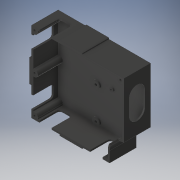
# Autodesk Inventor part: electronics_compartement
Saved by Autodesk Inventor 2019.4 (Build 234330000, 330)
## iProperties
Created: 2020-10-28
Part Number: electronics_compartement
Material: Generic
Document SubType Name: Modeling
Designer: deanv
Density: 1 g/cm^3
Appearance: Smooth - Black
Author: deanv
Autodesk Inventor part; units mm, degrees
ref_plane "YZ Plane" through (0, 0, 0) normal (1, 0, 0) x (0, 1, 0)
ref_plane "XZ Plane" through (0, 0, 0) normal (0, 1, 0) x (-1, 0, 0)
ref_plane "XY Plane" through (0, 0, 0) normal (0, 0, 1) x (1, 0, 0)
sketch "Sketch1" plane through (0, 0, 0) normal (0, 0, 1) x (1, 0, 0)
  line L0 (-73.5, 64) -> (73.5, 64)
  line L1 (73.5, 64) -> (73.5, -64)
  line L2 (73.5, -64) -> (-73.5, -64)
  line L3 (-73.5, -64) -> (-73.5, 64)
  line L4 (-73.5, 64) -> (73.5, -64) construction
  line L5 (73.5, 64) -> (-73.5, -64) construction
  line L6 (71, -61.5) -> (-71, -61.5)
  line L7 (-71, -61.5) -> (-71, 61.5)
  line L8 (-71, 61.5) -> (71, 61.5)
  line L9 (71, 61.5) -> (71, -61.5)
  line L10 (71, -61.5) -> (-71, 61.5) construction
  line L11 (-71, -61.5) -> (71, 61.5) construction
  line L12 (-73.5, 18.5) -> (-76.5, 18.5)
  line L13 (-76.5, 18.5) -> (-76.5, -18.5)
  line L14 (-76.5, -18.5) -> (-73.5, -18.5)
  line L15 (-73.5, -18.5) -> (-73.5, 18.5)
  line L16 (-73.5, 0) -> (73.5, 0) construction
  line L17 (0, -64) -> (0, 64) construction
  line L18 (-28.5, 64) -> (7.5, 64)
  line L19 (7.5, 64) -> (7.5, 66)
  line L20 (7.5, 66) -> (-28.5, 66)
  line L21 (-28.5, 66) -> (-28.5, 64)
  line L22 (-28.5, -64) -> (7.5, -64)
  line L23 (7.5, -64) -> (7.5, -66)
  line L24 (7.5, -66) -> (-28.5, -66)
  line L25 (-28.5, -66) -> (-28.5, -64)
  line L26 (73.5, -64) -> (51, -64) construction
  line L27 (51, -64) -> (51, -24.6) construction
  line L28 (51, -24.6) -> (73.5, -24.6) construction
  line L29 (73.5, -24.6) -> (73.5, -64) construction
  line L30 (51, -24.6) -> (73.5, -24.6) construction
  line L31 (73.5, -24.6) -> (73.5, -47.1) construction
  line L32 (73.5, -47.1) -> (51, -47.1) construction
  line L33 (51, -47.1) -> (51, -24.6) construction
  arc A0 (73.5, -24.6) -> (51, -47.1) centre (73.5, -47.1) ccw
  line L34 (51, -47.1) -> (51, -64)
  line L35 (73.5, -47.1) -> (48.5, -47.1) construction
  line L36 (48.5, -47.1) -> (48.5, -22.1) construction
  line L37 (48.5, -22.1) -> (73.5, -22.1) construction
  line L38 (73.5, -22.1) -> (73.5, -47.1) construction
  arc A1 (73.5, -22.1) -> (48.5, -47.1) centre (73.5, -47.1) ccw
  line L39 (48.5, -47.1) -> (48.5, -64)
  line L40 (-73.5, -64) -> (-68.5, -64) construction
  line L41 (-68.5, -64) -> (-68.5, -59) construction
  line L42 (-68.5, -59) -> (-73.5, -59) construction
  line L43 (-73.5, -59) -> (-73.5, -64) construction
  circle A2 centre (-68.5, -59) radius 5
  line L44 (-68.5, -54) -> (-73.5, -54)
  line L45 (-63.5, -59) -> (-63.5, -64)
  line L46 (-73.5, 64) -> (-68.5, 64) construction
  line L47 (-68.5, 64) -> (-68.5, 59) construction
  line L48 (-68.5, 59) -> (-73.5, 59) construction
  line L49 (-73.5, 59) -> (-73.5, 64) construction
  circle A3 centre (-68.5, 59) radius 5
  line L50 (-68.5, 54) -> (-73.5, 54)
  line L51 (-63.5, 59) -> (-63.5, 64)
  line L52 (-71, -1.25) -> (-68.5, -1.25) construction
  line L53 (-68.5, -1.25) -> (-68.5, 1.25) construction
  line L54 (-68.5, 1.25) -> (-71, 1.25) construction
  line L55 (-71, 1.25) -> (-71, -1.25) construction
  circle A4 centre (-68.5, 0) radius 5
  line L56 (-68.5, 5) -> (-73.5, 5)
  line L57 (-68.5, -5) -> (-73.5, -5)
  arc A5 (73.5, -24.6) -> (51, -47.1) centre (73.5, -47.1) ccw
  line L58 (51, -47.1) -> (51, -64)
  line L59 (51, -64) -> (73.5, -64)
  line L60 (73.5, -64) -> (73.5, -24.6)
  line L61 (71, 61.5) -> (-71, 61.5)
  line L62 (-71, 61.5) -> (-71, -61.5)
  line L63 (-71, -61.5) -> (71, -61.5)
  line L64 (71, -61.5) -> (71, 61.5)
  line L65 (71, 61.5) -> (-71, -61.5) construction
  line L66 (-71, 61.5) -> (71, -61.5) construction
  line L67 (73.5, 64) -> (-73.5, 64)
  line L68 (-73.5, 64) -> (-73.5, -64)
  line L69 (-73.5, -64) -> (73.5, -64)
  line L70 (73.5, -64) -> (73.5, 64)
  line L71 (73.5, 64) -> (-73.5, -64) construction
  line L72 (-73.5, 64) -> (73.5, -64) construction
  line L73 (-73.5, 64) -> (73.5, 64)
  line L74 (73.5, 64) -> (73.5, -64)
  line L75 (73.5, -64) -> (-73.5, -64)
  line L76 (-73.5, -64) -> (-73.5, 64)
  line L77 (71, -61.5) -> (-71, -61.5)
  line L78 (-71, -61.5) -> (-71, 61.5)
  line L79 (-71, 61.5) -> (71, 61.5)
  line L80 (71, 61.5) -> (71, -61.5)
  arc A6 (73.5, -24.6) -> (51, -47.1) centre (73.5, -47.1) ccw
  arc A7 (73.5, -22.1) -> (48.5, -47.1) centre (73.5, -47.1) ccw
  line L81 (73.5, -22.1) -> (73.5, -24.6)
  line L82 (51, -47.1) -> (51, -64)
  line L83 (51, -64) -> (48.5, -64)
  line L84 (48.5, -64) -> (48.5, -47.1)
  line L85 (73.5, 64) -> (68.5, 64) construction
  line L86 (68.5, 64) -> (68.5, 59) construction
  line L87 (68.5, 59) -> (73.5, 59) construction
  line L88 (73.5, 59) -> (73.5, 64) construction
  circle A8 centre (68.5, 59) radius 5
  line L89 (63.5, 59) -> (63.5, 64)
  line L90 (68.5, 54) -> (73.5, 54)
  circle A9 centre (17.2, 49) radius 3.25
  circle A10 centre (68, 33.777) radius 3.25
  circle A11 centre (68, 5.837) radius 3.25
  circle A12 centre (15.93, 0.757) radius 3.25
  circle A13 centre (17.2, 49) radius 3.25
  circle A14 centre (68, 33.777) radius 3.25
  circle A15 centre (68, 5.837) radius 3.25
  circle A16 centre (15.93, 0.757) radius 3.25
  line L91 (-33.5, -61.5) -> (16.5, -61.5) construction
  line L92 (16.5, -61.5) -> (16.5, 1.5) construction
  line L93 (16.5, 1.5) -> (-33.5, 1.5) construction
  line L94 (-33.5, 1.5) -> (-33.5, -61.5) construction
  line L95 (-33.5, -61.5) -> (16.5, 1.5) construction
  line L96 (16.5, -61.5) -> (-33.5, 1.5) construction
  line L97 (16.5, -51.5) -> (-33.5, -51.5) construction
  line L98 (-33.5, -51.5) -> (-33.5, -8.5) construction
  line L99 (-33.5, -8.5) -> (16.5, -8.5) construction
  line L100 (16.5, -8.5) -> (16.5, -51.5) construction
  line L101 (16.5, -51.5) -> (-33.5, -8.5) construction
  line L102 (-33.5, -51.5) -> (16.5, -8.5) construction
  line L103 (-8.5, 1.5) -> (-8.5, -61.5) construction
  circle A17 centre (-8.5, -4.5) radius 6
  circle A18 centre (-8.5, -55.5) radius 6
  point P0 (0, 0)
  point P1 (-8.5, -30)
  point P2 (0, -61.5)
  dimension "d130" = 12
  dimension "d131" = 12
  dimension "d0" = 147
  dimension "d1" = 128
  dimension "d7" = 37
  dimension "d8" = 18.5
  dimension "d9" = 3
  dimension "d10" = 2
  dimension "d11" = 36
  dimension "d12" = 45
  dimension "d13" = 2
  dimension "d14" = 36
  dimension "d15" = 45
  dimension "d16" = 22.5
  dimension "d17" = 39.4
  dimension "d18" = 22.5
  dimension "d19" = 22.5
  dimension "d20" = 142
  dimension "d21" = 123
  dimension "d22" = 25
  dimension "d23" = 25
  dimension "d24" = 25
  dimension "d25" = 5
  dimension "d26" = 5
  dimension "d27" = 5
  dimension "d28" = 5
  dimension "d29" = 2.5
  dimension "d30" = 2.5
  dimension "d31" = 1.25
  dimension "d92" = 5
  dimension "d93" = 5
  dimension "d105" = 27.94
  dimension "d106" = 52.07
  dimension "d107" = 48.243
  dimension "d108" = 50.8
  dimension "d109" = 1.27
  dimension "d110" = 5.08
  dimension "d111" = 3
  dimension "d112" = 12.5
  dimension "d113" = 6.5
  dimension "d114" = 6.5
  dimension "d115" = 6.5
  dimension "d116" = 6.5
  dimension "d126" = 63
  dimension "d127" = 50
  dimension "d128" = 50
  dimension "d129" = 43
  dimension "d132" = 37.5
  constraints: 208 end point, 37 parallel, 30 perpendicular, 21 point on circle, 20 midpoint, 18 horizontal, 17 centre point, 17 point on line, 13 coincident, 9 tangent, 7 concentric, 3 collinear, 2 vertical alignment, 4 other
  measures "d0" distance of L1.end L2.end
  measures "d1" distance of L0.end L1.end
  measures "d7" distance between parallel lines of L12 L14
  measures "d8" distance between parallel lines of L16 L12
  measures "d9" distance between parallel lines of L3 L13
  measures "d10" distance between parallel lines of L2 L24
  measures "d11" distance between parallel lines of L23 L25
  measures "d12" distance between parallel lines of L3 L25
  measures "d13" distance of L20.end L18.start
  measures "d14" distance of L19.end L20.end
  measures "d15" distance between parallel lines of L3 L21
  measures "d16" distance of L27.end L28.end
  measures "d17" distance of L26.end L27.end
  measures "d18" distance between parallel lines of L28 L32
  measures "d19" radius of A0
  measures "d20" distance of L6.start L6.end
  measures "d21" distance of L8.end L6.start
  measures "d22" distance of L36.end L37.end
  measures "d23" distance of L35.end L36.end
  measures "d24" radius of A1
  measures "d25" distance of L42.end L41.end
  measures "d26" distance of L41.end L40.end
  measures "d27" distance of L47.end L48.end
  measures "d28" distance of L46.end L47.end
  measures "d29" distance of L53.end L54.end
  measures "d30" distance of L52.end L53.end
  measures "d31" distance between parallel lines of L16 L54
  measures "d92" distance of L87.end L86.end
  measures "d93" distance of L86.end L85.end
  measures "d105" distance of point (68, 33.777) point (68, 5.837)
  measures "d106" horizontal distance of point (15.93, 0.757) point (68, 5.837)
  measures "d107" vertical distance of point (17.2, 49) point (15.93, 0.757)
  measures "d108" horizontal distance of point (68, 33.777) point (17.2, 49)
  measures "d109" horizontal distance of point (17.2, 49) point (15.93, 0.757)
  measures "d110" vertical distance of point (68, 5.837) point (15.93, 0.757)
  measures "d111" distance from line of L9 point (68, 5.837)
  measures "d112" distance from line of L8 point (17.2, 49)
  measures "d113" diameter of A9
  measures "d114" diameter of A10
  measures "d115" diameter of A11
  measures "d116" diameter of A12
  measures "d126" distance of L91.end L92.end
  measures "d127" distance of L91.start L91.end
  measures "d128" distance of L97.start L97.end
  measures "d129" distance between parallel lines of L99 L97
  measures "d132" distance between parallel lines of L78 L98
extrude "Extrusion1" add sketch "Sketch1" along normal blind 2.5 contours L0 L89 L8 L51 | A18 | L8 L89 A8 L90 L9 A10 A11 A1 L39 L6 L45 A2 L44 L7 L57 A4 L56 L50 A3 L51 | L89 L0 A8 L8 | L8 A8 L89 | L50 L7 L56 L3 | A8 L9 L8 | L8 L9 A8 | L0 L1 A8 | A8 L9 L90 | L1 L90 L9 A8 | L90 L1 A1 L9 A11 A10 | A10 L9 | L9 A10 | L1 A0 L9 A1 | L57 L7 L44 L3 | L1 L2 L34 L6 L9 A0 | L9 A0 L34 L6 L39 A1 | A11 L9 | L9 A11 | L9 L6 L34 A0 | L2 L39 L6 L34 | L39 L2 L45 L6 | A9 | A12 | A17
extrude "Extrusion2" add sketch "Sketch1" along normal blind 45 contours L21 L20 L19 L0 | L3 L14 L13 L12 | L56 L7 A4 L3 | L56 A4 L7 | A4 L7 L57 L3 | A4 L7 | A4 L7 | A4 L57 L7 | L23 L24 L25 L2
extrude "Extrusion3" add sketch "Sketch1" along normal blind 45 contours L44 L7 A2 L3 | L44 A2 L7 | A2 L2 L3 | A2 L7 L6 | A2 L6 L7 | A2 L6 L45 L2 | L45 L6 A2
extrude "Extrusion4" add sketch "Sketch1" along normal blind 45 contours L51 L8 A3 L0 | A3 L3 L0 | A3 L8 L7 | L51 A3 L8 | A3 L7 L8 | A3 L7 L50 L3 | A3 L50 L7
extrude "Extrusion5" cut sketch "Sketch1" along normal blind 45 contours L1 L2 L34 L6 L9 A0 | L9 L6 L34 A0
extrude "Extrusion6" add sketch "Sketch1" along normal blind 45 contours L51 L8 A3 L0 | L0 L89 L8 L51 | A3 L3 L0 | A3 L8 L7 | L51 A3 L8 | A18 | L8 L89 A8 L90 L9 A10 A11 A1 L39 L6 L45 A2 L44 L7 L57 A4 L56 L50 A3 L51 | A3 L7 L8 | A3 L7 L50 L3 | L89 L0 A8 L8 | L8 A8 L89 | L50 L7 L56 L3 | A3 L50 L7 | A8 L9 L8 | L8 L9 A8 | L0 L1 A8 | A8 L9 L90 | L1 L90 L9 A8 | L56 L7 A4 L3 | L56 A4 L7 | L90 L1 A1 L9 A11 A10 | A4 L7 L57 L3 | A4 L7 | A4 L7 | A10 L9 | L9 A10 | L1 A0 L9 A1 | L57 L7 L44 L3 | A4 L57 L7 | L1 L2 L34 L6 L9 A0 | L9 A0 L34 L6 L39 A1 | L44 L7 A2 L3 | A11 L9 | L9 A11 | L9 L6 L34 A0 | L44 A2 L7 | A2 L2 L3 | A2 L7 L6 | L2 L39 L6 L34 | L39 L2 L45 L6 | A2 L6 L7 | A2 L6 L45 L2 | L45 L6 A2 | A9 | A12 | A17
extrude "Extrusion7" cut sketch "Sketch1" along normal blind 45 contours L51 A3 L8 | A18 | L8 L89 A8 L90 L9 A10 A11 A1 L39 L6 L45 A2 L44 L7 L57 A4 L56 L50 A3 L51 | A3 L7 L8 | L8 A8 L89 | A3 L50 L7 | L8 L9 A8 | A8 L9 L90 | L56 A4 L7 | A4 L7 | L9 A10 | A4 L57 L7 | L9 A0 L34 L6 L39 A1 | L9 A11 | L9 L6 L34 A0 | L44 A2 L7 | A2 L6 L7 | L45 L6 A2 | A9 | A12 | A17 picked at (-66.9911, 57.4911) picked at (66.9911, 57.4911) picked at (-68.2785, 0.4936) picked at (68.0388, 32.7494) picked at (68.5933, 5.512) picked at (-66.9911, -57.4911)
extrude "Extrusion8" add sketch "Sketch1" along normal blind 2.5 contours L51 L8 A3 L0 | L0 L89 L8 L51 | A3 L3 L0 | A3 L8 L7 | L51 A3 L8 | A18 | L8 L89 A8 L90 L9 A10 A11 A1 L39 L6 L45 A2 L44 L7 L57 A4 L56 L50 A3 L51 | A3 L7 L8 | A3 L7 L50 L3 | L89 L0 A8 L8 | L8 A8 L89 | L50 L7 L56 L3 | A3 L50 L7 | A8 L9 L8 | L8 L9 A8 | L0 L1 A8 | A8 L9 L90 | L1 L90 L9 A8 | L56 L7 A4 L3 | L56 A4 L7 | L90 L1 A1 L9 A11 A10 | A4 L7 L57 L3 | A4 L7 | A4 L7 | A10 L9 | L9 A10 | L1 A0 L9 A1 | L57 L7 L44 L3 | A4 L57 L7 | L1 L2 L34 L6 L9 A0 | L9 A0 L34 L6 L39 A1 | L44 L7 A2 L3 | A11 L9 | L9 A11 | L9 L6 L34 A0 | L44 A2 L7 | A2 L2 L3 | A2 L7 L6 | L2 L39 L6 L34 | L39 L2 L45 L6 | A2 L6 L7 | A2 L6 L45 L2 | L45 L6 A2 | A9 | A12 | A17
extrude "Extrusion9" add sketch "Sketch1" along normal blind 45 contours L44 L7 A2 L3 | L44 A2 L7 | A2 L2 L3 | A2 L7 L6 | A2 L6 L7 | A2 L6 L45 L2 | L45 L6 A2
extrude "Extrusion10" add sketch "Sketch1" along normal blind 45 contours L51 L8 A3 L0 | A3 L3 L0 | A3 L8 L7 | L51 A3 L8 | A3 L7 L8 | A3 L7 L50 L3 | A3 L50 L7 | L3 L14 L13 L12 | L56 L7 A4 L3 | L56 A4 L7 | A4 L7 L57 L3 | A4 L7 | A4 L7 | A4 L57 L7
extrude "Extrusion11" cut sketch "Sketch1" along normal blind 45 contours L1 L2 L34 L6 L9 A0 | L9 L6 L34 A0
extrude "Extrusion12" add sketch "Sketch1" along normal blind 45 contours L1 A0 L9 A1 | L9 A0 L34 L6 L39 A1 | L2 L39 L6 L34
sketch "Sketch2" plane through (0, 0, 45) normal (0, 0, 1) x (1, 0, 0)
  arc A0 (73.5, -24.6) -> (51, -47.1) centre (73.5, -47.1) ccw projected
  line L0 (73.5, -24.6) -> (73.5, 64) projected
  line L1 (73.5, 64) -> (7.5, 64) projected
  line L2 (7.5, 64) -> (7.5, 66) projected
  line L3 (7.5, 66) -> (-28.5, 66) projected
  line L4 (-28.5, 66) -> (-28.5, 64) projected
  line L5 (-28.5, 64) -> (-73.5, 64) projected
  line L6 (-73.5, 64) -> (-73.5, 18.5) projected
  line L7 (-73.5, 18.5) -> (-76.5, 18.5) projected
  line L8 (-76.5, 18.5) -> (-76.5, -18.5) projected
  line L9 (-76.5, -18.5) -> (-73.5, -18.5) projected
  line L10 (-73.5, -18.5) -> (-73.5, -64) projected
  line L11 (-73.5, -64) -> (-28.5, -64) projected
  line L12 (-28.5, -64) -> (-28.5, -66) projected
  line L13 (-28.5, -66) -> (7.5, -66) projected
  line L14 (7.5, -66) -> (7.5, -64) projected
  line L15 (7.5, -64) -> (51, -64) projected
  line L16 (51, -64) -> (51, -47.1) projected
  arc A1 (71, -22.2253) -> (48.5, -47.1) centre (73.5, -47.1) ccw projected
  line L17 (48.5, -47.1) -> (48.5, -61.5) projected
  line L18 (48.5, -61.5) -> (-63.5, -61.5) projected
  line L19 (-63.5, -61.5) -> (-63.5, -59) projected
  arc A2 (-63.5, -59) -> (-68.5, -54) centre (-68.5, -59) ccw projected
  line L20 (-68.5, -54) -> (-71, -54) projected
  line L21 (-71, -54) -> (-71, -5) projected
  line L22 (-71, -5) -> (-68.5, -5) projected
  arc A3 (-68.5, -5) -> (-68.5, 5) centre (-68.5, 0) ccw projected
  line L23 (-68.5, 5) -> (-71, 5) projected
  line L24 (-71, 5) -> (-71, 54) projected
  line L25 (-71, 54) -> (-68.5, 54) projected
  arc A4 (-68.5, 54) -> (-63.5, 59) centre (-68.5, 59) ccw projected
  line L26 (-63.5, 59) -> (-63.5, 61.5) projected
  line L27 (-63.5, 61.5) -> (71, 61.5) projected
  line L28 (71, 61.5) -> (71, -22.2253) projected
  arc A5 (73.5, -24.6) -> (51, -47.1) centre (73.5, -47.1) ccw projected
  line L29 (73.5, -24.6) -> (73.5, 64) projected
  line L30 (73.5, 64) -> (7.5, 64) projected
  line L31 (7.5, 64) -> (7.5, 66) projected
  line L32 (7.5, 66) -> (-28.5, 66) projected
  line L33 (-28.5, 66) -> (-28.5, 64) projected
  line L34 (-28.5, 64) -> (-73.5, 64) projected
  line L35 (-73.5, 64) -> (-73.5, 18.5) projected
  line L36 (-73.5, 18.5) -> (-76.5, 18.5) projected
  line L37 (-76.5, 18.5) -> (-76.5, -18.5) projected
  line L38 (-76.5, -18.5) -> (-73.5, -18.5) projected
  line L39 (-73.5, -18.5) -> (-73.5, -64) projected
  line L40 (-73.5, -64) -> (-28.5, -64) projected
  line L41 (-28.5, -64) -> (-28.5, -66) projected
  line L42 (-28.5, -66) -> (7.5, -66) projected
  line L43 (7.5, -66) -> (7.5, -64) projected
  line L44 (7.5, -64) -> (51, -64) projected
  line L45 (51, -64) -> (51, -47.1) projected
  arc A6 (71, -22.2253) -> (48.5, -47.1) centre (73.5, -47.1) ccw projected
  line L46 (48.5, -47.1) -> (48.5, -61.5) projected
  line L47 (48.5, -61.5) -> (-63.5, -61.5) projected
  line L48 (-63.5, -61.5) -> (-63.5, -59) projected
  arc A7 (-63.5, -59) -> (-68.5, -54) centre (-68.5, -59) ccw projected
  line L49 (-68.5, -54) -> (-71, -54) projected
  line L50 (-71, -54) -> (-71, -5) projected
  line L51 (-71, -5) -> (-68.5, -5) projected
  arc A8 (-68.5, -5) -> (-68.5, 5) centre (-68.5, 0) ccw projected
  line L52 (-68.5, 5) -> (-71, 5) projected
  line L53 (-71, 5) -> (-71, 54) projected
  line L54 (-71, 54) -> (-68.5, 54) projected
  arc A9 (-68.5, 54) -> (-63.5, 59) centre (-68.5, 59) ccw projected
  line L55 (-63.5, 59) -> (-63.5, 61.5) projected
  line L56 (-63.5, 61.5) -> (71, 61.5) projected
  line L57 (71, 61.5) -> (71, -22.2253) projected
  line L58 (-73.5, 64) -> (-28.5, 64) construction
  line L59 (-28.5, 64) -> (-28.5, 19) construction
  line L60 (-28.5, 19) -> (-73.5, 19) construction
  line L61 (-73.5, 19) -> (-73.5, 64) construction
  line L62 (-73.5, -64) -> (-28.5, -64) construction
  line L63 (-28.5, -64) -> (-28.5, -19) construction
  line L64 (-28.5, -19) -> (-73.5, -19) construction
  line L65 (-73.5, -19) -> (-73.5, -64) construction
  line L66 (-73.5, 31.5) -> (-71, 31.5)
  line L67 (-71, 31.5) -> (-71, 51.5)
  line L68 (-71, 51.5) -> (-73.5, 51.5)
  line L69 (-73.5, 51.5) -> (-73.5, 31.5)
  line L70 (-63.5, 61.5) -> (71, 61.5) projected
  line L71 (-61, 64) -> (-41, 64)
  line L72 (-41, 64) -> (-41, 61.5)
  line L73 (-41, 61.5) -> (-61, 61.5)
  line L74 (-61, 61.5) -> (-61, 64)
  line L75 (-73.5, -51.5) -> (-71, -51.5)
  line L76 (-71, -51.5) -> (-71, -31.5)
  line L77 (-71, -31.5) -> (-73.5, -31.5)
  line L78 (-73.5, -31.5) -> (-73.5, -51.5)
  line L79 (-61, -61.5) -> (-41, -61.5)
  line L80 (-41, -61.5) -> (-41, -64)
  line L81 (-41, -64) -> (-61, -64)
  line L82 (-61, -64) -> (-61, -61.5)
  line L83 (20, -64) -> (40, -64)
  line L84 (40, -64) -> (40, -61.5)
  line L85 (40, -61.5) -> (20, -61.5)
  line L86 (20, -61.5) -> (20, -64)
  line L87 (73.5, -47.1) -> (48.5, -47.1) construction
  line L88 (48.5, -47.1) -> (48.5, -22.1) construction
  line L89 (48.5, -22.1) -> (73.5, -22.1) construction
  line L90 (73.5, -22.1) -> (73.5, -47.1) construction
  line L91 (73.5, -47.1) -> (48.5, -22.1) construction
  line L92 (66.4289, -54.1711) -> (41.4289, -29.1711)
  line L93 (41.4289, -29.1711) -> (55.5711, -15.0289)
  line L94 (55.5711, -15.0289) -> (80.5711, -40.0289)
  line L95 (80.5711, -40.0289) -> (66.4289, -54.1711)
  line L96 (66.4289, -54.1711) -> (55.5711, -15.0289) construction
  line L97 (41.4289, -29.1711) -> (80.5711, -40.0289) construction
  line L98 (73.5, 64) -> (68.5, 64) construction
  line L99 (68.5, 64) -> (68.5, 59) construction
  line L100 (68.5, 59) -> (73.5, 59) construction
  line L101 (73.5, 59) -> (73.5, 64) construction
  point P0 (0, 0)
  point P1 (61, -34.6)
  dimension "d58" = 45
  dimension "d59" = 45
  dimension "d60" = 45
  dimension "d61" = 45
  dimension "d62" = 20
  dimension "d63" = 20
  dimension "d64" = 20
  dimension "d65" = 20
  dimension "d66" = 12.5
  dimension "d67" = 12.5
  dimension "d68" = 12.5
  dimension "d69" = 20
  dimension "d70" = 12.5
  dimension "d73" = 25
  dimension "d74" = 25
  dimension "d75" = 20
  dimension "d76" = 35.3553
  dimension "d96" = 5
  dimension "d97" = 5
  constraints: 86 end point, 21 parallel, 11 point on line, 10 perpendicular, 9 horizontal, 4 coincident, 3 midpoint
  measures "d58" distance of L59.end L60.end
  measures "d59" distance of L58.end L59.end
  measures "d60" distance of L63.end L64.end
  measures "d61" distance of L62.end L63.end
  measures "d62" distance between parallel lines of L72 L74
  measures "d63" distance between parallel lines of L66 L68
  measures "d64" distance between parallel lines of L77 L75
  measures "d65" distance between parallel lines of L80 L82
  measures "d66" distance between parallel lines of L6 L74
  measures "d67" distance between parallel lines of L5 L68
  measures "d68" distance between parallel lines of L40 L75
  measures "d69" distance between parallel lines of L84 L86
  measures "d70" distance between parallel lines of L14 L86
  measures "d73" distance of L88.end L89.end
  measures "d74" distance of L87.end L88.end
  measures "d75" distance of L92.end L93.end
  measures "d76" distance between parallel lines of L93 L95
  measures "d96" distance of L100.end L99.end
  measures "d97" distance of L99.end L98.end
extrude "Extrusion13" cut sketch "Sketch2" against normal blind 2.5 contours A0 L94 A1 L28 L27 L72 L5 L4 L3 L2 L1 L0 | A0 L92 A1 L94 | A0 L16 L15 L84 L18 L17 A1 L92 | L15 L86 L18 L84 | L27 L74 L5 L72 | L15 L14 L13 L12 L11 L80 L18 L86 | L27 L26 A4 L25 L24 L68 L6 L5 L74 | L80 L11 L82 L18 | L82 L11 L10 L75 L21 L20 A2 L19 L18 | L68 L24 L66 L6 | L66 L24 L23 A3 L22 L21 L77 L10 L9 L8 L7 L6 | L10 L77 L21 L75
extrude "Extrusion14" cut sketch "Sketch2" against normal blind 35 contours L15 L86 L18 L84 | L27 L74 L5 L72 | L80 L11 L82 L18 | L68 L24 L66 L6 | L10 L77 L21 L75
extrude "Extrusion15" cut sketch "Sketch2" against normal blind 35 contours L94 L95 L92 A0 | A0 L92 A1 L94 | A1 L92 L93 L94
fillet "Fillet1" radius 5 12 edges at (-72.25, -31.5, 10) (-72.25, -51.5, 10) (-61, -62.75, 10) (-41, -62.75, 10) (20, -62.75, 10) (40, -62.75, 10) (51.2019, -38.944, 10) (65.344, -24.8019, 10) (-72.25, 51.5, 10) (-72.25, 31.5, 10) (-41, 62.75, 10) (-61, 62.75, 10)
hole "Hole1" at (-68.5, -59, 45) at (-68.5, 0, 45) at (-68.5, 59, 45) direction (0, 0, -1) diameter 4 depth 8
sketch "Sketch3" plane through (73.5, -24.6, 0) normal (1, 0, 0) x (0, 0, -1)
  line L0 (-42.5, 0) -> (0, 0) construction
  line L1 (0, 0) -> (0, 88.6) construction
  line L2 (0, 88.6) -> (-42.5, 88.6) construction
  line L3 (-42.5, 88.6) -> (-42.5, 0) construction
  line L4 (-42.5, 88.6) -> (-42.5, 86.1) construction
  line L5 (0, 0) -> (-42.5, 88.6) construction
  line L6 (0, 88.6) -> (0, 43.1) construction
  line L7 (-42.5, 0) -> (0, 88.6) construction
  line L8 (-21.25, 56.8) -> (-21.25, 31.8) construction
  line L9 (0, 43.1) -> (-42.5, 43.1) projected
  line L10 (-33.75, 56.8) -> (-33.75, 31.8)
  line L11 (-8.75, 31.8) -> (-8.75, 56.8)
  arc A0 (-8.75, 56.8) -> (-33.75, 56.8) centre (-21.25, 56.8) ccw
  arc A1 (-33.75, 31.8) -> (-8.75, 31.8) centre (-21.25, 31.8) ccw
  line L12 (-21.25, 44.3) -> (3.75, 44.3) construction
  point P0 (0, 24.6)
  dimension "d87" = 12.5
  dimension "d88" = 90
  dimension "d89" = 25
  constraints: 22 end point, 4 point on circle, 4 tangent, 3 parallel, 3 perpendicular, 2 centre point, 2 horizontal, 2 midpoint
  measures "d87" distance of L12.start L8.end
  measures "d88" angle of L8 L12
  measures "d89" diameter of A1
extrude "Extrusion16" cut sketch "Sketch3" against normal blind 35
extrude "Extrusion17" add sketch "Sketch1" along normal blind 42.5 contours L89 L0 A8 L8 | L8 A8 L89 | A8 L9 L8 | L8 L9 A8 | L0 L1 A8 | A8 L9 L90 | L1 L90 L9 A8
hole "Hole2" at (68.5, 59, 45) direction (0, 0, -1) diameter 4 depth 8
extrude "Extrusion18" add sketch "Sketch1" along normal blind 5 contours A10 L9 | L9 A10 | A11 L9 | L9 A11 | A9 | A12
hole "Hole3" at (68, 33.777, 0) at (68, 5.837, 0) at (17.2, 49, 0) at (15.93, 0.757, 0) direction (0, 0, 1) diameter 3 depth 5 counterbore diameter 5.5 counterbore depth 3
extrude "Extrusion19" add sketch "Sketch1" along normal blind 5 contours A18 | A17
hole "Hole4" at (-8.5, -4.5, 0) at (-8.5, -55.5, 0) direction (0, 0, 1) diameter 4 depth 5 counterbore diameter 8.5 counterbore depth 4
equation "\"d131\" = d130"
equation "\"d8\" = 0.5 * d7"
equation "\"d13\" = d10"
equation "\"d14\" = d11"
equation "\"d15\" = d12"
equation "\"d18\" = d16"
equation "\"d23\" = d22"
equation "\"d26\" = d25"
equation "\"d27\" = d26"
equation "\"d28\" = d27"
equation "\"d29\" = 0.5 * d28"
equation "\"d30\" = d29"
equation "\"d31\" = 0.5 * d30"
equation "\"d114\" = d113"
equation "\"d115\" = d114"
equation "\"d116\" = d115"
equation "\"d128\" = d127"
equation "\"d59\" = d58"
equation "\"d60\" = d58"
equation "\"d61\" = d60"
equation "\"d63\" = d62"
equation "\"d64\" = d63"
equation "\"d65\" = d64"
equation "\"d66\" = d67"
equation "\"d68\" = d66"
equation "\"d69\" = d65"
equation "\"d70\" = d67"
body "Solid1"
